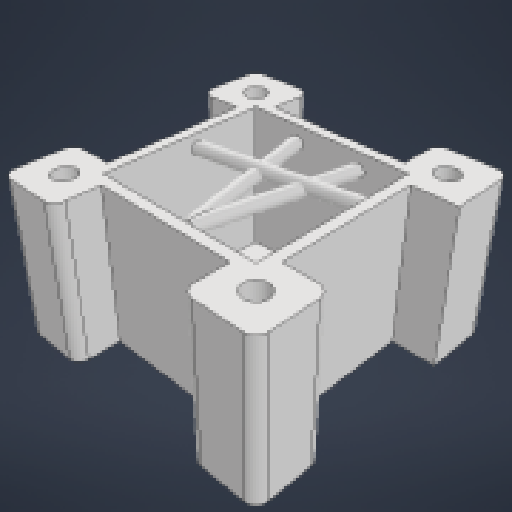
# Autodesk Inventor part: Huevo
Saved by Autodesk Inventor 2026.1 (Build 301233000, 233)
## iProperties
Created: 2025-11-15
Part Number: Huevo
Material: PLA
Document SubType Name: Modeling
Designer: vickh
Density: 1.29 g/cm^3
Appearance: Genérico
Mass: 227.145 g
Surface Area: 616.798 cm^2
Volume: 176.082 cm^3
Author: vickh
Autodesk Inventor part; units mm, degrees
ref_plane "YZ Plane" through (0, 0, 0) normal (1, 0, 0) x (0, 1, 0)
ref_plane "XZ Plane" through (0, 0, 0) normal (0, 1, 0) x (-1, 0, 0)
ref_plane "XY Plane" through (0, 0, 0) normal (0, 0, 1) x (1, 0, 0)
sketch "Boceto1" plane through (0, 0, 0) normal (0, 1, 0) x (-1, 0, 0)
  line L0 (25, 33.5) -> (-25, 33.5)
  line L1 (33.5, -25) -> (33.5, 25)
  circle A0 centre (0, 0) radius 5 construction
  line L2 (-33.5, 25) -> (-33.5, -25)
  line L3 (-25, -33.5) -> (25, -33.5)
  line L4 (-25, -49) -> (-25, -33.5)
  line L5 (-33.5, -25) -> (-49, -25)
  line L6 (-49, -25) -> (-49, -49)
  line L7 (-49, -49) -> (-25, -49)
  line L8 (-49, 25) -> (-33.5, 25)
  line L9 (-49, 49) -> (-49, 25)
  line L10 (-25, 49) -> (-49, 49)
  line L11 (-25, 33.5) -> (-25, 49)
  line L12 (33.5, 25) -> (49, 25)
  circle A1 centre (37, 37) radius 4.15
  line L13 (49, 25) -> (49, 49)
  line L14 (49, 49) -> (25, 49)
  line L15 (25, 49) -> (25, 33.5)
  line L16 (49, -49) -> (49, -25)
  line L17 (49, -25) -> (33.5, -25)
  line L18 (25, -49) -> (49, -49)
  line L19 (25, -33.5) -> (25, -49)
  line L20 (49, -49) -> (-49, -49) construction
  line L21 (-49, -49) -> (-49, 49)
  line L22 (-49, 49) -> (49, 49) construction
  line L23 (49, 49) -> (49, -49) construction
  line L24 (49, -49) -> (19.5933, -49) construction
  line L25 (0, -49) -> (0, 49) construction
  line L26 (49, 0) -> (-49, 0) construction
  line L27 (49, 49) -> (25, 49) construction
  line L28 (25, 49) -> (25, 25) construction
  line L29 (25, 25) -> (49, 25) construction
  line L30 (49, 25) -> (49, 49) construction
  line L31 (49, 49) -> (25, 25) construction
  line L32 (49, 25) -> (25, 49) construction
  circle A2 centre (-37, 37) radius 4.15
  circle A3 centre (-37, -37) radius 4.15
  circle A4 centre (37, -37) radius 4.15
  line L33 (29.5, 29.5) -> (-29.5, 29.5)
  line L34 (-29.5, 29.5) -> (-29.5, -29.5)
  line L35 (-29.5, -29.5) -> (29.5, -29.5)
  line L36 (29.5, -29.5) -> (29.5, 29.5)
  line L37 (29.5, 29.5) -> (-29.5, -29.5) construction
  line L38 (-29.5, 29.5) -> (29.5, -29.5) construction
  circle A5 centre (0, 0) radius 2.5 construction
  point P0 (33.5, 0)
  point P1 (0, -33.5)
  point P2 (0, 33.5)
  point P3 (-33.5, 0)
  dimension "d2" = 33.5
  dimension "d3" = 33.5
  dimension "d4" = 8.3
  dimension "d5" = 49
  dimension "d6" = 49
  dimension "d7" = 98
  dimension "d8" = 98
  dimension "d9" = 15.5
  dimension "d10" = 15.5
  dimension "d11" = 15.5
  dimension "d12" = 15.5
  dimension "d13" = 50
  dimension "d14" = 50
  dimension "d15" = 15.5
  dimension "d16" = 15.5
  dimension "d17" = 15.5
  dimension "d18" = 50
  dimension "d19" = 25
  dimension "d20" = 25
  dimension "d21" = 25
  dimension "d22" = 25
  dimension "d23" = 10
  dimension "d24" = 8.5
  dimension "d25" = 8.5
  dimension "d26" = 24
  dimension "d27" = 15.5
  dimension "d28" = 24
  dimension "d29" = 8.5
  dimension "d30" = 24
  dimension "d31" = 24
  dimension "d32" = 360
  dimension "d33" = 4
  dimension "d34" = 5
  dimension "d35" = 4
  constraints: 78 end point, 11 midpoint, 7 horizontal, 7 vertical, 6 centre point, 6 parallel, 4 coincident, 3 perpendicular, 3 point on line, 9 other
  measures "d2" distance of point (0, 0) point (33.5, 0)
  measures "d3" distance from line of point (0, 0) L2
  measures "d4" diameter of A1
  measures "d5" distance of point (0, 0) L26.end
  measures "d6" distance from line of L20 point (0, 0)
  measures "d7" distance of L20.start L20.end
  measures "d8" distance of L20.end L22.start
  measures "d9" distance between parallel lines of L22 L0
  measures "d10" distance between parallel lines of L23 L1
  measures "d11" distance between parallel lines of L20 L3
  measures "d12" distance of L2.end L5.end
  measures "d13" distance of L4.end L19.start
  measures "d14" distance of L0.start L0.end
  measures "d15" distance of L14.end L0.start
  measures "d16" distance of L0.end L11.end
  measures "d17" distance of L8.start L2.start
  measures "d18" distance of L2.start L2.end
  measures "d19" distance from line of point (0, 0) L5
  measures "d20" distance from line of L17 point (0, 0)
  measures "d21" distance from line of point (0, 0) L12
  measures "d22" distance from line of point (0, 0) L8
  measures "d23" diameter of A0
  measures "d24" horizontal distance of L2.end L4.end
  measures "d25" distance from line of L11 L2.start
  measures "d26" distance of L12.end L13.end
  measures "d27" distance of L4.start L4.end
  measures "d28" distance of L13.end L14.end
  measures "d29" horizontal distance of L1.start L19.start
  measures "d30" distance of L29.end L29.start
  measures "d31" distance of L29.start L27.end
  measures "d33" distance between parallel lines of L35 L3
  measures "d34" diameter of A5
  measures "d35" distance between parallel lines of L1 L36
extrude "Extrusión1" add sketch "Boceto1" along normal blind 55 contours L15 L14 L13 L12 L1 L17 L16 L18 L19 L3 L4 L7 L6 L5 L2 L8 L9 L10 L11 L0
extrude "Extrusión2" add sketch "Boceto1" along normal blind 4 contours L36 L35 L34 L33
sketch "Boceto2" plane through (29.5, 55, 29.5) normal (0, 0, -1) x (-1, 0, 0)
  line L0 (0, -51) -> (59, -51) projected
  line L1 (59, 0) -> (0, 0)
  line L2 (0, 0) -> (0, -51)
  line L3 (0, -51) -> (59, -51)
  line L4 (59, -51) -> (59, 0)
  line L5 (0, -51) -> (0, 0) construction
  line L6 (59, 0) -> (0, -51) construction
  line L7 (0, 0) -> (59, -51) construction
  line L8 (29.5, 0) -> (29.5, -51) construction
  line L9 (59, -25.5) -> (0, -25.5) construction
  line L10 (59, -51) -> (0, -51)
  line L11 (0, -51) -> (0, -39)
  line L12 (0, -39) -> (59, -39) construction
  line L13 (59, -39) -> (59, -51)
  line L14 (59, -45) -> (0, -45) construction
  circle A0 centre (6.9412, -45) radius 2.5
  circle A1 centre (52.0588, -45) radius 2.5
  line L15 (0, 0) -> (59, 0)
  line L16 (59, 0) -> (59, -12)
  line L17 (59, -12) -> (0, -12)
  line L18 (0, -12) -> (0, 0)
  line L19 (0, -6) -> (59, -6) construction
  point P0 (29.5, -55)
  point P1 (29.5, -25.5)
  dimension "d40" = 12
  dimension "d41" = 5
  dimension "d42" = 5
  dimension "d58" = 12
  constraints: 36 end point, 9 midpoint, 6 parallel, 5 point on line, 4 horizontal, 3 perpendicular, 2 centre point, 1 collinear
  measures "d40" distance between parallel lines of L12 L0
  measures "d41" diameter of A0
  measures "d42" diameter of A1
  measures "d58" distance of L15.end L16.end
sketch "Boceto3" plane through (-29.5, 55, -29.5) normal (0, 0, 1) x (1, 0, 0)
  line L0 (59, -51) -> (59, 0) projected
  line L1 (0, -51) -> (59, -51)
  line L2 (59, -51) -> (59, 0)
  line L3 (59, 0) -> (0, 0)
  line L4 (0, 0) -> (0, -51)
  line L5 (0, -51) -> (59, -51)
  line L6 (59, -51) -> (59, -38)
  line L7 (59, -38) -> (0, -38)
  line L8 (0, -38) -> (0, -51)
  line L9 (54.5, -55) -> (4.5, -55) projected
  line L10 (0, -51) -> (0, 0) construction
  line L11 (0, -51) -> (59, 0) construction
  line L12 (59, -51) -> (0, 0) construction
  line L13 (0, -44.5) -> (59, -44.5) construction
  line L14 (0, 0) -> (59, 0) construction
  line L15 (29.5, 0) -> (29.5, -51) construction
  line L16 (0, 0) -> (59, 0)
  line L17 (59, 0) -> (59, -12)
  line L18 (59, -12) -> (0, -12)
  line L19 (0, -12) -> (0, 0)
  line L20 (0, -6) -> (59, -6)
  circle A0 centre (17.5, -6) radius 2.5
  circle A1 centre (41.5, -6) radius 2.5
  point P0 (29.5, -55)
  point P1 (29.5, -55)
  point P2 (29.5, -6)
  dimension "d50" = 13
  dimension "d60" = 12
  dimension "d61" = 5
  dimension "d62" = 5
  dimension "d63" = 12
  dimension "d64" = 12
  constraints: 34 end point, 8 midpoint, 6 parallel, 3 horizontal, 3 perpendicular, 3 point on line, 2 centre point, 1 collinear
  measures "d50" distance between parallel lines of L1 L7
  measures "d60" distance of L16.end L17.end
  measures "d61" diameter of A0
  measures "d62" diameter of A1
  measures "d63" distance of point (29.5, -6) A0.centre
  measures "d64" distance of point (29.5, -6) A1.centre
sketch "Boceto4" plane through (0, 4, 0) normal (0, 1, 0) x (1, 0, 0)
  line L0 (-29.5, 29.5) -> (29.5, 29.5) projected
  line L1 (-22.5588, -29.5) -> (8, 29.5)
  point P0 (0, 0)
  point P1 (0, 29.5)
  point P2 (0, 29.5)
  point P3 (0, 29.5)
  point P4 (22.5588, -29.5)
  point P5 (0, 29.5)
  dimension "d56" = 8
  constraints: 2 end point, 1 midpoint, 1 point on line
  measures "d56" distance of point (0, 29.5) L1.end
sweep "Barrido1" add profiles "Boceto2" path "Boceto4" path curves L1 contours A1
sketch "Boceto5" plane through (0, 4, 0) normal (0, 1, 0) x (1, 0, 0)
  line L0 (-29.5, 29.5) -> (29.5, 29.5) projected
  line L1 (-29.5, 29.5) -> (29.5, 29.5) projected
  line L2 (22.5588, -29.5) -> (-8, 29.5)
  point P0 (0, 0)
  point P1 (0, 29.5)
  point P2 (0, 29.5)
  point P3 (0, 29.5)
  point P4 (0, 29.5)
  dimension "d57" = 8
  constraints: 2 end point, 1 midpoint, 1 point on line
  measures "d57" distance of L2.end point (0, 29.5)
sweep "Barrido2" add profiles "Boceto2" path "Boceto5" path curves L2 contours A0
sketch "Boceto6" plane through (-29.5, 55, 29.5) normal (1, 0, 0) x (0, 0, -1)
  line L0 (0, 0) -> (59, 0)
  line L1 (59, 0) -> (59, -51)
  line L2 (59, -51) -> (0, -51)
  line L3 (0, -51) -> (0, 0)
  line L4 (0, -51) -> (59, -51)
  line L5 (59, -51) -> (59, -39)
  line L6 (59, -39) -> (0, -39) construction
  line L7 (0, -39) -> (0, -51)
  line L8 (0, -39) -> (59, -51) construction
  line L9 (0, -51) -> (0, 0) construction
  line L10 (0, -51) -> (59, -39) construction
  line L11 (0, -51) -> (59, -51) projected
  line L12 (59, -51) -> (59, 0) projected
  line L13 (0, -51) -> (59, -51)
  line L14 (59, -51) -> (59, -44.5)
  line L15 (0, -44.5) -> (0, -51)
  circle A0 centre (9.5, -45) radius 2.5
  line L16 (29.5, -45) -> (0, -45)
  point P0 (29.5, -55)
  point P1 (59, -38)
  point P2 (59, -38)
  point P3 (59, -38)
  dimension "d49" = 12
  dimension "d51" = 6.5
  dimension "d52" = 5
  dimension "d53" = 20
  constraints: 28 end point, 5 parallel, 4 perpendicular, 4 point on line, 3 horizontal, 1 centre point, 1 midpoint
  measures "d49" distance between parallel lines of L2 L6
  measures "d51" distance of L14.end L13.end
  measures "d52" diameter of A0
  measures "d53" distance of L16.start A0.centre
sketch "Boceto7" plane through (0, 4, 0) normal (0, 1, 0) x (1, 0, 0)
  line L0 (29.5, 29.5) -> (29.5, -29.5) projected
  line L1 (-29.5, -20) -> (29.5, -15)
  line L2 (29.5, 29.5) -> (29.5, -29.5) projected
  point P0 (0, 0)
  point P1 (29.5, 0)
  dimension "d79" = 15
  constraints: 2 end point, 1 midpoint, 1 point on line
  measures "d79" distance of L1.end point (29.5, 0)
sweep "Barrido3" add profiles "Boceto6" path "Boceto7" path curves L1 contours L16 A0 | A0 L16
sketch "Boceto8" plane through (0, 4, 0) normal (0, 1, 0) x (1, 0, 0)
  line L0 (29.5, -29.5) -> (-29.5, -29.5) projected
  line L1 (29.5, -29.5) -> (-29.5, -29.5) projected
  line L2 (-12, 29.5) -> (1, -29.5)
  point P0 (0, 0)
  point P1 (12, 29.5)
  point P2 (0, -29.5)
  dimension "d65" = 1
  constraints: 2 end point, 1 midpoint, 1 point on line
  measures "d65" distance of point (0, -29.5) L2.end
sweep "Barrido4" add profiles "Boceto3" path "Boceto8" path curves L2 contours A0 L20 | L20 A0
sketch "Boceto9" plane through (0, 4, 0) normal (0, 1, 0) x (1, 0, 0)
  line L0 (29.5, -29.5) -> (-29.5, -29.5) projected
  line L1 (29.5, -29.5) -> (-29.5, -29.5) projected
  line L2 (12, 29.5) -> (-1, -29.5)
  point P0 (0, 0)
  point P1 (0, -29.5)
  dimension "d68" = 1
  constraints: 2 end point, 1 midpoint, 1 point on line
  measures "d68" distance of point (0, -29.5) L2.end
sweep "Barrido5" add profiles "Boceto3" path "Boceto9" path curves L2 contours A1 L20 | L20 A1
sketch "Boceto10" plane through (29.5, 55, -29.5) normal (-1, 0, 0) x (0, 0, 1)
  line L0 (0, -51) -> (0, 0) projected
  line L1 (0, 0) -> (59, 0)
  line L2 (59, 0) -> (59, -10)
  line L3 (59, -10) -> (0, -10)
  line L4 (0, -10) -> (0, 0)
  line L5 (59, -51) -> (59, 0) projected
  line L6 (0, -10) -> (59, 0)
  line L7 (59, -10) -> (0, 0)
  line L8 (0, -5) -> (59, -5)
  circle A0 centre (14.5, -5) radius 2.5
  point P0 (29.5, -55)
  point P1 (29.5, 0)
  point P2 (29.5, -5)
  dimension "d71" = 10
  dimension "d72" = 5
  dimension "d73" = 15
  constraints: 14 end point, 3 midpoint, 2 parallel, 2 perpendicular, 2 point on line, 1 centre point, 1 collinear, 1 horizontal
  measures "d71" distance from line of L3 point (29.5, 0)
  measures "d72" diameter of A0
  measures "d73" distance of point (29.5, -5) A0.centre
sketch "Boceto11" plane through (-29.5, 55, 29.5) normal (1, 0, 0) x (0, 0, -1)
  line L0 (59, -51) -> (59, 0) projected
  line L1 (59, 0) -> (0, 0)
  line L2 (0, 0) -> (0, -13)
  line L3 (0, -13) -> (59, -13)
  line L4 (59, -13) -> (59, 0)
  line L5 (0, -51) -> (0, 0) projected
  line L6 (59, 0) -> (0, -13)
  line L7 (0, 0) -> (59, -13)
  line L8 (59, -6.5) -> (0, -6.5)
  circle A0 centre (34.5, -6.5) radius 3
  point P0 (29.5, -55)
  point P1 (29.5, -6.5)
  dimension "d74" = 13
  dimension "d75" = 6
  dimension "d76" = 5
  constraints: 14 end point, 2 midpoint, 2 parallel, 2 perpendicular, 2 point on line, 1 centre point, 1 collinear, 1 horizontal
  measures "d74" distance between parallel lines of L1 L3
  measures "d75" diameter of A0
  measures "d76" distance of point (29.5, -6.5) A0.centre
sketch "Boceto12" plane through (0, 4, 0) normal (0, 1, 0) x (1, 0, 0)
  line L0 (29.5, 15) -> (-29.5, 5)
  point P0 (0, 0)
  constraints: 2 end point
sweep "Barrido6" add profiles "Boceto10" path "Boceto12" separate body contours A0 L8 | L8 A0
fillet "Empalme1" radius 4 12 edges at (49, 27.5, -49) (25, 27.5, -49) (-25, 27.5, -49) (-49, 27.5, -49) (-49, 27.5, -25) (-49, 27.5, 25) (-49, 27.5, 49) (-25, 27.5, 49) (49, 27.5, 49) (49, 27.5, 25) (25, 27.5, 49) (49, 27.5, -25)
chamfer "Chaflán1" distance 4 angle 45 8 edges at (-25, 27.5, 33.5) (25, 27.5, 33.5) (33.5, 27.5, 25) (33.5, 27.5, -25) (25, 27.5, -33.5) (-25, 27.5, -33.5) (-33.5, 27.5, -25) (-33.5, 27.5, 25)
equation "\"d57\" = d56"
equation "\"d68\" = d65"
